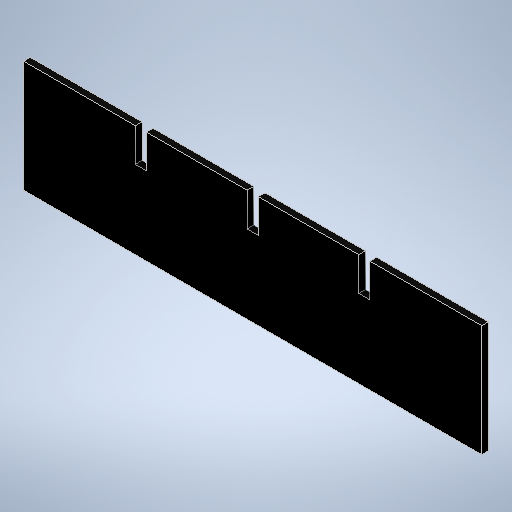
# Autodesk Inventor part: Sensors Shield
Saved by Autodesk Inventor 2025.4 (Build 294407000, 407)
## iProperties
Created: 2026-04-19
Part Number: Sensors Shield
Material: Generic
Document SubType Name: Sheet Metal
Designer: lenovo
Density: 1 g/cm^3
Sheet Metal Rule: Default_mm
Appearance: Default(1)
Author: lenovo
Autodesk Inventor part; units mm, degrees
ref_plane "YZ Plane" through (0, 0, 0) normal (1, 0, 0) x (0, 1, 0)
ref_plane "XZ Plane" through (0, 0, 0) normal (0, 1, 0) x (-1, 0, 0)
ref_plane "XY Plane" through (0, 0, 0) normal (0, 0, 1) x (1, 0, 0)
sketch "Sketch1" plane through (0, 0, 0) normal (0, 0, 1) x (1, 0, 0)
  line L0 (-102.5, -25) -> (102.5, -25)
  line L1 (102.5, -25) -> (102.5, 25)
  line L2 (102.5, 25) -> (-102.5, 25)
  line L3 (-102.5, 25) -> (-102.5, -25)
  line L4 (-102.5, -25) -> (102.5, 25) construction
  line L5 (102.5, -25) -> (-102.5, 25) construction
  point P0 (0, 0)
  dimension "d0" = 205
  dimension "d1" = 50
  measures "d0" distance of L2.end L1.end
  measures "d1" distance of L1.end L0.end
extrude "Plate1" add sketch "Sketch1" along normal blind 3
sketch "Sketch2" plane through (0, 0, 3) normal (0, 0, 1) x (1, 0, 0)
  line L0 (102.5, 25) -> (-102.5, 25) projected
  line L1 (47.5, 25) -> (52.5, 25)
  line L2 (52.5, 25) -> (52.5, 10)
  line L3 (52.5, 10) -> (47.5, 10)
  line L4 (47.5, 10) -> (47.5, 25)
  line L5 (102.5, 25) -> (102.5, -25) projected
  point P0 (0, 0)
  point P1 (52.5, 25)
  dimension "d3" = 50
  dimension "d4" = 5
  dimension "d5" = 15
  constraints: 8 end point, 2 parallel, 1 horizontal, 1 perpendicular, 1 point on line
  measures "d3" distance between parallel lines of L2 L5
  measures "d4" distance between parallel lines of L2 L4
  measures "d5" distance of L3.end L1.start
extrude "Cut1" cut sketch "Sketch2" against normal blind 3
pattern_linear "Rectangular Pattern1" count 3 spacing 50 along (-1, 0, 0) of "Cut1"
equation "\"d6\" = Thickness"
equation "\"d2\" = Thickness"
equation "\"BendRadius\" = Thickness"
equation "\"BendReliefWidth\" = Thickness"
equation "\"BendReliefDepth\" = 0.5 * Thickness"
equation "\"CornerReliefSize\" = 4 * Thickness"
equation "\"MinimumRemnant\" = 2 * Thickness"
equation "\"TransitionRadius\" = BendRadius"
equation "\"JacobiRadiusSize\" = BendRadius"
equation "\"GapSize\" = Thickness"
equation "\"Thickness\" = 3"
body "Solid1"
